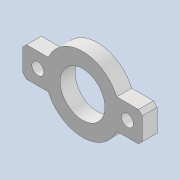
# Autodesk Inventor part: bearing_holder_2
Saved by Autodesk Inventor 2020 (Build 240168000, 168)
## iProperties
Created: 2021-07-19
Part Number: bearing_holder_2
Material: Generic
Document SubType Name: Modeling
Designer: Shuang Peng
Density: 1 g/cm^3
Appearance: Default
Author: Shuang Peng
Autodesk Inventor part; units mm, degrees
ref_plane "YZ Plane" through (0, 0, 0) normal (1, 0, 0) x (0, 1, 0)
ref_plane "XZ Plane" through (0, 0, 0) normal (0, 1, 0) x (-1, 0, 0)
ref_plane "XY Plane" through (0, 0, 0) normal (0, 0, 1) x (1, 0, 0)
sketch "Sketch1" plane through (0, 0, 0) normal (0, 0, 1) x (1, 0, 0)
  circle A0 centre (0, 0) radius 5
  line L0 (8.5, -2) -> (8.5, 2)
  line L1 (8.5, 2) -> (-8.5, 2)
  line L2 (-8.5, 2) -> (-8.5, -2)
  line L3 (-8.5, -2) -> (8.5, -2)
  line L4 (8.5, -2) -> (-8.5, 2) construction
  line L5 (8.5, 2) -> (-8.5, -2) construction
  point P0 (4.5826, 2)
  point P1 (-4.5826, 2)
  point P2 (-4.5826, -2)
  point P3 (4.5826, -2)
  dimension "d0" = 10
  dimension "d1" = 4
  dimension "d2" = 17
  constraints: 12 end point, 2 midpoint, 2 parallel, 1 centre point, 1 coincident, 1 perpendicular, 1 vertical
  measures "d0" diameter of A0
  measures "d1" distance of L0.start L0.end
  measures "d2" distance of L1.end L0.end
extrude "Extrusion1" add sketch "Sketch1" along normal blind 2
sketch "Sketch2" plane through (0, 0, 0) normal (0, 0, -1) x (-1, 0, 0)
  circle A0 centre (-6, 0) radius 0.8 projected
  circle A1 centre (6, 0) radius 0.8 projected
  circle A2 centre (0, 0) radius 2.25 projected
  line L0 (15, 2) -> (4.5826, 2) projected
  arc A3 (4.5826, 2) -> (-4.5826, 2) centre (0, 0) ccw projected
  line L1 (-4.5826, 2) -> (-15, 2) projected
  line L2 (-15, 2) -> (-15, -2) projected
  line L3 (-15, -2) -> (-4.5826, -2) projected
  arc A4 (-4.5826, -2) -> (4.5826, -2) centre (0, 0) ccw projected
  line L4 (4.5826, -2) -> (15, -2) projected
  line L5 (15, -2) -> (15, 2) projected
hole "Hole1" at (6, 0, 0) at (-6, 0, 0) direction (0, 0, 1) diameter 1.6 end through all
sketch "Sketch3" plane through (0, 0, 0) normal (0, 0, -1) x (-1, 0, 0)
  circle A0 centre (0, 0) radius 3
  dimension "d12" = 6
  constraints: 1 centre point, 1 coincident
  measures "d12" diameter of A0
extrude "Extrusion2" cut sketch "Sketch3" against normal blind 2
thicken "Thicken1" operation add thickness 0.5 both sides no extend neighbours yes toward (1, 0, 0) faces at (-8.5, 0.6667, 0.6667)
thicken "Thicken2" operation add thickness 0.5 both sides no extend neighbours yes toward (-1, 0, 0) faces at (8.5, -0.6667, 0.6667)
chamfer "Chamfer1" distance 0.5 angle 45 4 edges at (8, -2, 1) (8, 2, 1) (-8, -2, 1) (-8, 2, 1)
body "Solid1"
